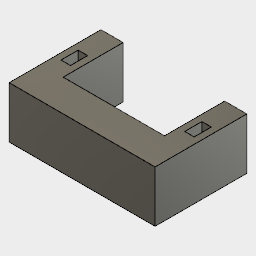
Bearing Case v15 (Autodesk Fusion 360 design; units mm, degrees)
Autodesk Fusion 360 part; units mm, degrees
sketch "Sketch1" plane through (0, 0, 0) normal (0, 1, 0) x (1, 0, 0)
  line L0 (-50, 15) -> (35, 15)
  line L1 (35, 15) -> (35, -15)
  line L2 (35, -15) -> (-50, -15)
  line L3 (-50, -15) -> (-50, 15)
  dimension "d1" = 85
  dimension "d2" = 30
  measures "d1" distance of L0.start L0.end
  measures "d2" distance of L0.start L2.end
extrude "Extrude1" add sketch "Sketch1" along normal blind 15 makes body 1
sketch "Sketch2" plane through (0, 0, 0) normal (0, 1, 0) x (1, 0, 0)
  line L0 (-50, 15) -> (-35, 15)
  line L1 (-35, 15) -> (-35, -15)
  line L2 (-35, -15) -> (-50, -15)
  line L3 (-50, -15) -> (-50, 15)
  point P0 (-50, 15)
  dimension "d5" = 15
  measures "d5" distance of P0 L0.end
extrude "Extrude2" add sketch "Sketch2" along normal blind 50 bodies 1
sketch "Sketch3" plane through (0, 0, 0) normal (0, 1, 0) x (1, 0, 0)
  line L0 (35, 15) -> (22, 15)
  line L1 (22, 15) -> (22, -15)
  line L2 (22, -15) -> (35, -15)
  line L3 (35, -15) -> (35, 15)
  line L4 (-35, 15) -> (-37, 15)
  line L5 (-37, 15) -> (-37, -15)
  line L6 (-37, -15) -> (-35, -15)
  line L7 (-35, -15) -> (-35, 15)
  point P0 (35, 15)
  point P1 (-35, 15)
  dimension "d8" = 13
  dimension "d9" = 2
  measures "d8" distance of P0 L0.end
  measures "d9" distance of P1 L4.end
extrude "Extrude3" cut sketch "Sketch3" along normal blind 50 contours L4 L5 L6 L7 bodies 1 makes body 2 at (-11.6667, 0, -5)
sketch "Sketch4" plane through (0, 0, 15) normal (0, 0, 1) x (1, 0, 0)
  line L0 (-35, 15) -> (-35, 0)
  line L1 (-35, 0) -> (35, 0)
  line L2 (35, 0) -> (35, 15)
  line L3 (35, 15) -> (-35, 15)
sketch "Sketch5" plane through (0, 0, 0) normal (0, 1, 0) x (1, 0, 0)
  line L0 (-35, -15) -> (-37, -15)
  line L1 (-37, -15) -> (-37, 15)
  line L2 (-37, 15) -> (-35, 15)
  line L3 (-35, 15) -> (-35, -15)
  point P0 (-35, -15)
  point P1 (-37, 15)
extrude "Extrude4" add sketch "Sketch5" along normal blind 15 bodies 1 2
extrude "Extrude5" add sketch "Sketch3" along normal blind 50 contours L0 L1 L2 L3 bodies 1
sketch "Sketch9" plane through (0, 0, 0) normal (0, -1, 0) x (1, 0, 0)
  line L0 (35, 15) -> (-50, 15)
  line L1 (-50, 15) -> (-50, -15)
  line L2 (-50, -15) -> (35, -15)
  line L3 (35, -15) -> (35, 15)
  line L4 (-50, 15) -> (35, 15)
  line L5 (35, 15) -> (35, -15)
  line L6 (35, -15) -> (-50, -15)
  line L7 (-50, -15) -> (-50, 15)
extrude "Extrude8" add 1 faces at (-21.6667, 0, -5) along direction (0, -1, 0) blind 3.5 on bodies 1 bodies 1
move_body "Move1" bodies 1 to x (1, 0, 0) y (0, 1, 0) z (0, 0, 1) at (0, 3.5, 0)
sketch "Sketch6" plane through (0, 0, 15) normal (0, 0, 1) x (1, 0, 0)
  line L0 (22, 18.5) -> (-37, 18.5)
  line L1 (-37, 18.5) -> (-37, 53.5)
  line L2 (-37, 53.5) -> (-50, 53.5)
  line L3 (-50, 53.5) -> (-50, 0)
  line L4 (35, 0) -> (35, 53.5)
  line L5 (35, 53.5) -> (22, 53.5)
  line L6 (22, 53.5) -> (22, 18.5)
  line L7 (-46.25, 36.5) -> (-40.75, 36.5)
  line L8 (-40.75, 36.5) -> (-40.75, 26.5)
  line L9 (-40.75, 26.5) -> (-46.25, 26.5)
  line L10 (-46.25, 26.5) -> (-46.25, 36.5)
  line L11 (31.25, 36.5) -> (31.25, 26.5)
  line L12 (31.25, 26.5) -> (25.75, 26.5)
  line L13 (25.75, 36.5) -> (31.25, 36.5)
  line L14 (25.75, 26.5) -> (25.75, 36.5)
  line L15 (-50, 0) -> (35, 0)
  dimension "d16" = 5.5
  dimension "d17" = 10
  dimension "d18" = 5.5
  dimension "d19" = 10
  measures "d16" distance of L7.start L7.end
  measures "d17" distance of L7.start L9.end
  measures "d18" distance of L13.start L11.start
  measures "d19" distance of L13.start L12.end
extrude "Extrude7" cut sketch "Sketch6" against normal blind 10.5 contours L11 L12 L13 L14 bodies 1
extrude "Extrude6" cut sketch "Sketch6" against normal blind 10.5 contours L7 L8 L9 L10 bodies 1
sketch "Sketch7" plane through (0, 0, 15) normal (0, 0, 1) x (1, 0, 0)
  line L0 (-40.75, 36.5) -> (-40.75, 26.5)
  line L1 (-40.75, 26.5) -> (-46.25, 26.5)
  line L2 (-46.25, 26.5) -> (-46.25, 36.5)
  line L3 (-46.25, 36.5) -> (-40.75, 36.5)
  line L4 (31.25, 36.5) -> (31.25, 26.5)
  line L5 (31.25, 26.5) -> (25.75, 26.5)
  line L6 (25.75, 26.5) -> (25.75, 36.5)
  line L7 (25.75, 36.5) -> (31.25, 36.5)
  line L8 (22, 18.5) -> (-37, 18.5)
  line L9 (-37, 18.5) -> (-37, 53.5)
  line L10 (-37, 53.5) -> (-50, 53.5)
  line L11 (-50, 53.5) -> (-50, 0)
  line L12 (35, 0) -> (35, 53.5)
  line L13 (35, 53.5) -> (22, 53.5)
  line L14 (22, 53.5) -> (22, 18.5)
  line L15 (-50, 0) -> (35, 0)
sketch "Sketch8" plane through (0, 0, 0) normal (0, 1, 0) x (1, 0, 0)
  line L0 (-50, 15) -> (35, 15)
  line L1 (35, 15) -> (35, -15)
  line L2 (35, -15) -> (-50, -15)
  line L3 (-50, -15) -> (-50, 15)
  line L4 (-50, 15) -> (35, 15)
  line L5 (35, 15) -> (35, -15)
  line L6 (35, -15) -> (-50, -15)
  line L7 (-50, -15) -> (-50, 15)
  line L8 (-50, 15) -> (35, 15)
  line L9 (35, 15) -> (35, -15)
  line L10 (35, -15) -> (-50, -15)
  line L11 (-50, -15) -> (-50, 15)
  line L12 (-50, 15) -> (35, 15)
  line L13 (35, 15) -> (35, -15)
  line L14 (35, -15) -> (-50, -15)
  line L15 (-50, -15) -> (-50, 15)
  point P0 (-50, 15)
  point P1 (35, -15)
  point P2 (-50, 15)
  point P3 (-50, 15)
move_body "Move2" bodies 1 to x (1, 0, 0) y (0, 0, -1) z (0, 1, 0) at (0, 0, 0)
move_body "Move3" bodies 1 to x (1, 0, 0) y (0, 1, 0) z (0, 0, 1) at (0, 15, 0)
